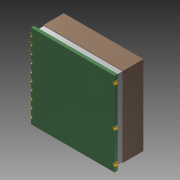
# Autodesk Inventor part: FGPMMOPA6C
Saved by Autodesk Inventor 2013 (Build 170138000, 138)
## iProperties
Created: 2015-07-03
Part Number: FGPMMOPA6C
Material: Ogólny
Document SubType Name: Modeling
Designer: terg
Density: 1 g/cm^3
Author: terg
Autodesk Inventor part; units mm, degrees
ref_plane "YZ Plane" through (0, 0, 0) normal (1, 0, 0) x (0, 1, 0)
ref_plane "XZ Plane" through (0, 0, 0) normal (0, 1, 0) x (-1, 0, 0)
ref_plane "XY Plane" through (0, 0, 0) normal (0, 0, 1) x (1, 0, 0)
sketch "Szkic1" plane through (0, 0, 0) normal (0, 1, 0) x (-1, 0, 0)
  line L0 (0, 0) -> (16, 0)
  line L1 (16, 0) -> (16, 16)
  line L2 (16, 16) -> (0, 16)
  line L3 (0, 16) -> (0, 0)
  dimension "d0" = 16
  dimension "d1" = 16
  constraints: 8 end point, 2 parallel, 1 horizontal, 1 perpendicular
  measures "d0" distance of L2.end L1.end
  measures "d1" distance of L1.end L0.end
extrude "Wyciągnięcie proste1" add sketch "Szkic1" along normal blind 0.6
sketch "Szkic2" plane through (0, 0.6, 0) normal (0, 1, 0) x (1, 0, 0)
  line L0 (0, 0) -> (-16, 0) projected
  line L1 (-16, 0) -> (-16, -16) projected
  line L2 (-16, -16) -> (0, -16) projected
  line L3 (0, -16) -> (0, 0) projected
  line L4 (-0.5, -0.5) -> (-15.5, -0.5)
  line L5 (-15.5, -0.5) -> (-15.5, -15.5)
  line L6 (-15.5, -15.5) -> (-0.5, -15.5)
  line L7 (-0.5, -15.5) -> (-0.5, -0.5)
  dimension "d4" = 15
  dimension "d5" = 15
  dimension "d6" = 0.5
  dimension "d7" = 0.5
  dimension "d8" = 0.5
  dimension "d9" = 0.5
  constraints: 8 end point, 2 parallel, 1 horizontal, 1 perpendicular
  measures "d4" distance of L6.end L5.end
  measures "d5" distance of L5.end L4.end
  measures "d6" distance between parallel lines of L4 L0
  measures "d7" distance between parallel lines of L2 L6
  measures "d8" distance between parallel lines of L1 L5
  measures "d9" distance between parallel lines of L3 L7
extrude "Wyciągnięcie proste2" add sketch "Szkic2" along normal blind 1.4 contours L7 L6 L5 L4
sketch "Szkic3" plane through (0, 2, 0) normal (0, 1, 0) x (1, 0, 0)
  line L0 (-0.5, -0.5) -> (-15.5, -0.5) projected
  line L1 (-15.5, -0.5) -> (-15.5, -15.5) projected
  line L2 (-15.5, -15.5) -> (-0.5, -15.5) projected
  line L3 (-0.5, -15.5) -> (-0.5, -0.5) projected
  line L4 (-15.6, -0.4) -> (-0.4, -0.4)
  line L5 (-0.4, -0.4) -> (-0.4, -15.6)
  line L6 (-0.4, -15.6) -> (-15.6, -15.6)
  line L7 (-15.6, -15.6) -> (-15.6, -0.4)
  point P0 (0, 0)
  dimension "d12" = 0.1
  dimension "d13" = 0.1
  dimension "d14" = 0.1
  dimension "d15" = 0.1
  constraints: 8 end point, 2 parallel, 1 horizontal, 1 perpendicular
  measures "d12" distance between parallel lines of L5 L3
  measures "d13" distance between parallel lines of L7 L1
  measures "d14" distance between parallel lines of L0 L4
  measures "d15" distance between parallel lines of L2 L6
extrude "Wyciągnięcie proste3" add sketch "Szkic3" along normal blind 4.2 contours L3 L2 L1 L0 | L4 L5 L6 L7
chamfer "Faza1" distance 0.3 angle 45 4 edges at (-15.6, 6.2, 8) (-8, 6.2, 0.4) (-0.4, 6.2, 8) (-8, 6.2, 15.6)
sketch "Szkic4" plane through (0, 6.2, 0) normal (0, 1, 0) x (1, 0, 0)
  line L0 (-0.7, -0.7) -> (-0.7, -15.3) projected
  line L1 (-15.3, -15.3) -> (-15.3, -0.7) projected
  line L2 (-0.7, -15.3) -> (-15.3, -15.3) projected
  line L3 (-13.25, -4.3) -> (-2.75, -4.3)
  line L4 (-2.75, -4.3) -> (-2.75, -13.25)
  line L5 (-2.75, -13.25) -> (-13.25, -13.25)
  line L6 (-13.25, -13.25) -> (-13.25, -4.3)
  point P0 (0, 0)
  dimension "d21" = 10.5
  dimension "d22" = 8.95
  dimension "d25" = 2.05
  dimension "d26" = 2.05
  dimension "d103" = 2.05
  constraints: 8 end point, 2 parallel, 1 horizontal, 1 perpendicular
  measures "d21" distance of L4.end L5.end
  measures "d22" distance of L3.end L4.end
  measures "d25" distance between parallel lines of L1 L6
  measures "d26" distance between parallel lines of L0 L4
  measures "d103" distance between parallel lines of L2 L5
extrude "Wyciągnięcie proste4" add sketch "Szkic4" along normal blind 0.01
sketch "Szkic5" plane through (0, 6.21, 0) normal (0, 1, 0) x (1, 0, 0)
  line L0 (-15, -4.3) -> (-1, -4.3)
  line L1 (-1, -4.3) -> (-1, -1.3)
  line L2 (-1, -1.3) -> (-15, -1.3)
  line L3 (-15, -1.3) -> (-15, -4.3)
  line L4 (-15.3, -15.3) -> (-15.3, -0.7) projected
  line L5 (-0.7, -0.7) -> (-0.7, -15.3) projected
  line L6 (-15.3, -0.7) -> (-0.7, -0.7) projected
  point P0 (0, 0)
  dimension "d29" = 14
  dimension "d31" = 3
  dimension "d32" = 0.3
  dimension "d33" = 0.3
  dimension "d34" = 0.6
  constraints: 8 end point, 2 parallel, 1 horizontal, 1 perpendicular
  measures "d29" distance of L2.end L1.end
  measures "d31" distance of L0.end L1.end
  measures "d32" distance between parallel lines of L4 L3
  measures "d33" distance between parallel lines of L5 L1
  measures "d34" distance between parallel lines of L6 L2
extrude "Wyciągnięcie proste5" add sketch "Szkic5" along normal blind 0.015
sketch "Szkic7" plane through (0, 6.2, 0) normal (0, 1, 0) x (1, 0, 0)
  line L0 (-0.7, -0.7) -> (-0.7, -15.3) projected
  line L1 (-15.3, -0.7) -> (-0.7, -0.7) projected
  line L2 (-15.3, -15.3) -> (-15.3, -0.7) projected
  line L3 (-0.7, -15.3) -> (-15.3, -15.3) projected
  circle A0 centre (-8, -8) radius 1.4
  circle A1 centre (-8, -8) radius 1.75
  point P0 (0, 0)
  dimension "d38" = 7.3
  dimension "d39" = 7.3
  dimension "d40" = 7.3
  dimension "d41" = 7.3
  dimension "d42" = 2.8
  dimension "d43" = 3.5
  constraints: 2 centre point, 2 coincident
  measures "d38" distance from line of L0 point (-8, -8)
  measures "d39" distance from line of L2 point (-8, -8)
  measures "d40" distance from line of L3 point (-8, -8)
  measures "d41" distance from line of L1 point (-8, -8)
  measures "d42" diameter of A0
  measures "d43" diameter of A1
extrude "Wyciągnięcie proste6" add sketch "Szkic7" along normal blind 0.015 contours A1
sketch "Szkic8" plane through (-8, 6.21, 8) normal (0, 1, 0) x (1, 0, 0)
  circle A0 centre (0, 0) radius 1.4 projected
  circle A1 centre (0, 0) radius 1.15
  point P0 (8, 8)
  dimension "d46" = 2.3
  constraints: 1 centre point, 1 coincident
  measures "d46" diameter of A1
extrude "Wyciągnięcie proste7" add sketch "Szkic8" along normal blind 0.4 contours A1
fillet "Zaokrąglenie1" radius 0.4 1 edges at (-9.15, 6.61, 8)
sketch "Szkic10" plane through (0, 0, 0) normal (0, -1, 0) x (1, 0, 0)
  line L0 (0, 0) -> (-16, 0) projected
  line L1 (0, 16) -> (0, 0) projected
  line L2 (-16, 16) -> (0, 16) projected
  line L3 (-16, 0) -> (-16, 16) projected
  point P0 (-16, 14.75)
  point P1 (-16, 13.25)
  point P2 (-16, 11.75)
  point P3 (-16, 10.25)
  point P4 (-16, 8.75)
  point P5 (-16, 7.25)
  point P6 (-16, 5.75)
  point P7 (-16, 4.25)
  point P8 (-16, 2.75)
  point P9 (-16, 1.25)
  point P10 (0, 1.25)
  point P11 (0, 14.75)
  point P12 (0, 7.25)
  dimension "d54" = 1.5
  dimension "d59" = 1.25
  dimension "d60" = 1.25
  dimension "d62" = 0
  dimension "d70" = 6
  dimension "d71" = 0
  constraints: 4 point on line, 1 vertical, 9 other
  measures "d54" distance of point (-16, 14.75) point (-16, 13.25)
  measures "d59" distance from line of L2 point (-16, 14.75)
  measures "d60" distance from line of L0 point (-16, 1.25)
  measures "d62" vertical distance of point (-16, 14.75) point (0, 14.75)
  measures "d70" distance of point (0, 1.25) point (0, 7.25)
  measures "d71" vertical distance of point (-16, 1.25) point (0, 1.25)
hole "Otwór1" at (-16, 0, 14.75) at (-16, 0, 13.25) at (-16, 0, 11.75) at (-16, 0, 10.25) at (-16, 0, 8.75) at (-16, 0, 7.25) at (-16, 0, 5.75) at (-16, 0, 4.25) at (-16, 0, 2.75) at (-16, 0, 1.25) at (0, 0, 1.25) at (0, 0, 14.75) at (0, 0, 7.25) direction (0, 1, 0) diameter 0.5 depth 8
sketch "Szkic11" plane through (0, 0, 0) normal (0, -1, 0) x (1, 0, 0)
  line L0 (-16, 1.5) -> (-16, 2.5) projected
  arc A0 (-16, 1) -> (-16, 1.5) centre (-16, 1.25) ccw projected
  line L1 (0, 1) -> (0, 0) projected
  arc A1 (0, 1.5) -> (0, 1) centre (0, 1.25) ccw projected
  line L2 (0, 7) -> (0, 1.5) projected
  line L3 (0, 14.5) -> (0, 7.5) projected
  arc A2 (-16.1, 0.9146) -> (-16.1, 1.5854) centre (-16, 1.25) ccw
  arc A3 (-16.1, 1.0209) -> (-16.1, 1.4791) centre (-16, 1.25) ccw
  line L4 (-16.1, 1.5854) -> (-16.1, 1.4791)
  line L5 (-16.1, 1.0209) -> (-16.1, 0.9146)
  arc A4 (-16.1, 2.4146) -> (-16.1, 3.0854) centre (-16, 2.75) ccw
  arc A5 (-16.1, 2.5209) -> (-16.1, 2.9791) centre (-16, 2.75) ccw
  line L6 (-16.1, 3.0854) -> (-16.1, 2.9791)
  line L7 (-16.1, 2.5209) -> (-16.1, 2.4146)
  arc A6 (-16.1, 3.9146) -> (-16.1, 4.5854) centre (-16, 4.25) ccw
  arc A7 (-16.1, 4.0209) -> (-16.1, 4.4791) centre (-16, 4.25) ccw
  line L8 (-16.1, 4.5854) -> (-16.1, 4.4791)
  line L9 (-16.1, 4.0209) -> (-16.1, 3.9146)
  arc A8 (-16.1, 5.4146) -> (-16.1, 6.0854) centre (-16, 5.75) ccw
  arc A9 (-16.1, 5.5209) -> (-16.1, 5.9791) centre (-16, 5.75) ccw
  line L10 (-16.1, 6.0854) -> (-16.1, 5.9791)
  line L11 (-16.1, 5.5209) -> (-16.1, 5.4146)
  arc A10 (-16.1, 6.9146) -> (-16.1, 7.5854) centre (-16, 7.25) ccw
  arc A11 (-16.1, 7.0209) -> (-16.1, 7.4791) centre (-16, 7.25) ccw
  line L12 (-16.1, 7.5854) -> (-16.1, 7.4791)
  line L13 (-16.1, 7.0209) -> (-16.1, 6.9146)
  arc A12 (-16.1, 8.4146) -> (-16.1, 9.0854) centre (-16, 8.75) ccw
  arc A13 (-16.1, 8.5209) -> (-16.1, 8.9791) centre (-16, 8.75) ccw
  line L14 (-16.1, 9.0854) -> (-16.1, 8.9791)
  line L15 (-16.1, 8.5209) -> (-16.1, 8.4146)
  arc A14 (-16.1, 9.9146) -> (-16.1, 10.5854) centre (-16, 10.25) ccw
  arc A15 (-16.1, 10.0209) -> (-16.1, 10.4791) centre (-16, 10.25) ccw
  line L16 (-16.1, 10.5854) -> (-16.1, 10.4791)
  line L17 (-16.1, 10.0209) -> (-16.1, 9.9146)
  arc A16 (-16.1, 11.4146) -> (-16.1, 12.0854) centre (-16, 11.75) ccw
  arc A17 (-16.1, 11.5209) -> (-16.1, 11.9791) centre (-16, 11.75) ccw
  line L18 (-16.1, 12.0854) -> (-16.1, 11.9791)
  line L19 (-16.1, 11.5209) -> (-16.1, 11.4146)
  arc A18 (-16.1, 12.9146) -> (-16.1, 13.5854) centre (-16, 13.25) ccw
  arc A19 (-16.1, 13.0209) -> (-16.1, 13.4791) centre (-16, 13.25) ccw
  line L20 (-16.1, 13.5854) -> (-16.1, 13.4791)
  line L21 (-16.1, 13.0209) -> (-16.1, 12.9146)
  arc A20 (-16.1, 14.4146) -> (-16.1, 15.0854) centre (-16, 14.75) ccw
  arc A21 (-16.1, 14.5209) -> (-16.1, 14.9791) centre (-16, 14.75) ccw
  line L22 (-16.1, 15.0854) -> (-16.1, 14.9791)
  line L23 (-16.1, 14.5209) -> (-16.1, 14.4146)
  arc A22 (0.1, 1.5854) -> (0.1, 0.9146) centre (0, 1.25) ccw
  arc A23 (0.1, 1.4791) -> (0.1, 1.0209) centre (0, 1.25) ccw
  line L24 (0.1, 1.4791) -> (0.1, 1.5854)
  line L25 (0.1, 1.0209) -> (0.1, 0.9)
  arc A24 (0.1, 7.5854) -> (0.1, 6.9146) centre (0, 7.25) ccw
  arc A25 (0.1, 7.4791) -> (0.1, 7.0209) centre (0, 7.25) ccw
  line L26 (0.1, 7.4791) -> (0.1, 7.5854)
  line L27 (0.1, 7.0209) -> (0.1, 6.9)
  arc A26 (0.1, 15.0854) -> (0.1, 14.4146) centre (0, 14.75) ccw
  arc A27 (0.1, 14.9791) -> (0.1, 14.5209) centre (0, 14.75) ccw
  line L28 (0.1, 14.9791) -> (0.1, 15.0854)
  line L29 (0.1, 14.5209) -> (0.1, 14.4)
  point P0 (-16, 3)
  point P1 (-16, 4.5)
  point P2 (-16, 4)
  point P3 (-16, 6)
  point P4 (-16, 5.5)
  point P5 (-16, 7.5)
  point P6 (-16, 7)
  point P7 (-16, 9)
  point P8 (-16, 8.5)
  point P9 (-16, 10.5)
  point P10 (-16, 10)
  point P11 (-16, 12)
  point P12 (-16, 11.5)
  point P13 (-16, 13.5)
  point P14 (-16, 13)
  point P15 (-16, 15)
  point P16 (-16, 14.5)
  point P17 (0, 7.5)
  point P18 (0, 13.5)
  point P19 (0, 14.5)
  point P20 (0, 15)
  dimension "d72" = 0.7
  dimension "d73" = 0.1
  dimension "d74" = 0.1
  dimension "d77" = 1.5
  dimension "d82" = 0.7
  dimension "d83" = 0.1
  dimension "d84" = 0.1
  dimension "d87" = 6
  dimension "d94" = 13.5
  constraints: 65 point on circle, 52 end point, 26 centre point, 26 coincident, 3 point on line, 3 vertical, 2 collinear, 2 parallel, 146 other
  measures "d72" diameter of A2
  measures "d73" distance between parallel lines of L0 L4
  measures "d74" distance from line of A0.start L5
  measures "d77" distance of A0.start point (-16, 2.5)
  measures "d82" diameter of A22
  measures "d83" distance between parallel lines of L2 L24
  measures "d84" distance between parallel lines of L1 L25
  measures "d87" distance of L1.start point (0, 7)
  measures "d94" distance of L2.end point (0, 15)
extrude "Wyciągnięcie proste8" add sketch "Szkic11" against normal blind 0.61 and the other way blind 0.01
equation "\"d6\" = d7"
equation "\"d8\" = d9"
equation "\"d25\" = d26"
equation "\"d32\" = d33"
equation "\"d38\" = d39"
equation "\"d40\" = d41"
equation "\"d59\" = d60"
